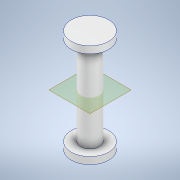
# Autodesk Inventor part: castshaft
Saved by Autodesk Inventor 2022 (Build 260153000, 153)
## iProperties
Created: 2022-04-20
Part Number: castshaft
Material: アルミニウム 6061
Document SubType Name: Modeling
Designer: Yazawa
Density: 2.7 g/cm^3
Appearance: アルミニウム - フラット
Author: Yazawa
Autodesk Inventor part; units mm, degrees
ref_plane "YZ Plane" through (0, 0, 0) normal (1, 0, 0) x (0, 1, 0)
ref_plane "XZ Plane" through (0, 0, 0) normal (0, 1, 0) x (-1, 0, 0)
ref_plane "XY Plane" through (0, 0, 0) normal (0, 0, 1) x (1, 0, 0)
sketch "スケッチ1" plane through (0, 0, 0) normal (0, 0, 1) x (1, 0, 0)
  line L0 (0, 11) -> (-4, 11)
  line L1 (-4, 11) -> (-4, 9.5)
  line L2 (-4, 9.5) -> (-2, 9.5)
  line L3 (-2, 9.5) -> (-2, 0)
  line L4 (-2, 0) -> (0, 0)
  line L5 (0, 0) -> (0, 11)
  line L6 (0, -2.2) -> (0, 13.2) projected
  dimension "d0" = 4
  dimension "d1" = 1.5
  dimension "d2" = 2
  dimension "d3" = 11
  constraints: 12 end point, 5 perpendicular, 1 horizontal
  measures "d0" distance of L0.start L0.end
  measures "d1" distance of L0.end L1.end
  measures "d2" distance between parallel lines of L5 L3
  measures "d3" distance of L4.end L0.start
revolve "回転1" add sketch "スケッチ1" angle 360 about axis through (0, -10, 0) along (0, 1, 0)
mirror "ミラー1" about plane through (-2, 0, 0) normal (0, -1, 0) of "回転1"
ref_plane "作業平面1" through (0, 0, 0) normal (0, -1, 0) x (1, 0, 0)
